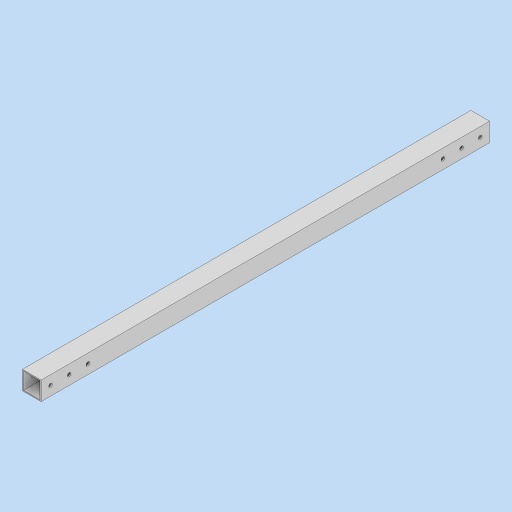
# Autodesk Inventor part: 24in long 1in square tube
Saved by Autodesk Inventor 2024 (Build 280153000, 153)
## iProperties
Created: 2024-01-10
Part Number: 24in long 1in square tube
Material: Generic
Document SubType Name: Modeling
Designer: david
Density: 1 g/cm^3
Appearance: Default
Author: david
Autodesk Inventor part; units mm, degrees
ref_plane "YZ Plane" through (0, 0, 0) normal (1, 0, 0) x (0, 1, 0)
ref_plane "XZ Plane" through (0, 0, 0) normal (0, 1, 0) x (-1, 0, 0)
ref_plane "XY Plane" through (0, 0, 0) normal (0, 0, 1) x (1, 0, 0)
sketch "Sketch1" plane through (0, 0, 0) normal (0, 0, 1) x (1, 0, 0)
  line L0 (-12.7, -12.7) -> (-12.7, 12.7)
  line L1 (-12.7, 12.7) -> (12.7, 12.7)
  line L2 (12.7, 12.7) -> (12.7, -12.7)
  line L3 (12.7, -12.7) -> (-12.7, -12.7)
  line L4 (-12.7, -12.7) -> (12.7, 12.7) construction
  line L5 (-12.7, 12.7) -> (12.7, -12.7) construction
  line L6 (11.1125, 11.1125) -> (-11.1125, 11.1125)
  line L7 (-11.1125, 11.1125) -> (-11.1125, -11.1125)
  line L8 (-11.1125, -11.1125) -> (11.1125, -11.1125)
  line L9 (11.1125, -11.1125) -> (11.1125, 11.1125)
  point P0 (0, 0)
  dimension "d0" = 25.4
  dimension "d1" = 25.4
  dimension "d2" = 1.5875
  constraints: 20 end point, 4 parallel, 2 midpoint, 2 perpendicular, 1 vertical, 3 other
  measures "d0" distance of L0.end L1.end
  measures "d1" distance of L1.end L2.end
  measures "d2" distance between parallel lines of L1 L6
extrude "Extrusion1" add sketch "Sketch1" along normal blind 609.6
sketch "Sketch2" plane through (12.7, -12.7, 0) normal (1, 0, 0) x (0, 0, -1)
  line L0 (0, 0) -> (0, 25.4) projected
  line L1 (0, 25.4) -> (-609.6, 25.4) projected
  line L2 (-609.6, 0) -> (-609.6, 25.4) projected
  line L3 (0, 0) -> (-609.6, 0) projected
  circle A0 centre (-596.9, 12.7) radius 2.5781
  circle A1 centre (-571.5, 12.7) radius 2.5781
  circle A2 centre (-546.1, 12.7) radius 2.5781
  line L4 (-304.8, 0) -> (-304.8, 25.4) construction
  circle A3 centre (-12.7, 12.7) radius 2.5781
  circle A4 centre (-38.1, 12.7) radius 2.5781
  circle A5 centre (-63.5, 12.7) radius 2.5781
  point P0 (0, 12.7)
  dimension "d5" = 5.1562
  dimension "d7" = 12.7
  dimension "d8" = 25.4
  dimension "d9" = 25.4
  constraints: 6 centre point, 3 symmetric about line, 2 end point, 2 midpoint, 1 equal radius, 3 other
  measures "d5" diameter of A0
  measures "d7" distance from line of A0.centre L2
  measures "d8" distance of A1.centre A0.centre
  measures "d9" distance of A2.centre A1.centre
extrude "Extrusion2" cut sketch "Sketch2" against normal through all contours A0 | A1 | A2 | A3 | A4 | A5
equation "\"d1\" = d0"
body "Solid1"
